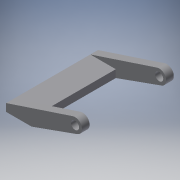
# Autodesk Inventor part: FiberMount
Saved by Autodesk Inventor 2019 (Build 230136000, 136)
## iProperties
Created: 2019-05-24
Part Number: FiberMount
Material: Generic
Document SubType Name: Modeling
Designer: aorfi
Density: 1 g/cm^3
Appearance: Default
Author: aorfi
Autodesk Inventor part; units mm, degrees
ref_plane "YZ Plane" through (0, 0, 0) normal (1, 0, 0) x (0, 1, 0)
ref_plane "XZ Plane" through (0, 0, 0) normal (0, 1, 0) x (-1, 0, 0)
ref_plane "XY Plane" through (0, 0, 0) normal (0, 0, 1) x (1, 0, 0)
sketch "Sketch1" plane through (0, 0, 0) normal (0, 1, 0) x (-1, 0, 0)
  line L0 (-5, 15) -> (5, 15)
  line L1 (5, 15) -> (5, -15)
  line L2 (5, -15) -> (-5, -15)
  line L3 (-5, -15) -> (-5, 15)
  line L4 (-5, 15) -> (5, -15) construction
  line L5 (5, 15) -> (-5, -15) construction
  point P0 (0, 0)
  dimension "d0" = 30
  dimension "d1" = 10
  constraints: 12 end point, 2 midpoint, 2 parallel, 1 horizontal, 1 perpendicular
  measures "d0" distance of L0.end L1.end
  measures "d1" distance of L1.end L2.end
extrude "Extrusion1" add sketch "Sketch1" along normal mid plane 3
sketch "Sketch2" plane through (-5, 1.5, 15) normal (0, 0, 1) x (1, 0, 0)
  circle A0 centre (27, 6) radius 1.5875
  circle A1 centre (27, 6) radius 2.75
  line L0 (26.1395, 8.6119) -> (0, 0)
  line L1 (10, -3) -> (10, 0) projected
  line L2 (10, -3) -> (27.926, 3.4106)
  line L3 (10, -3) -> (0, -3) projected
  line L4 (0, 0) -> (0, -3) projected
  point P0 (5, -1.5)
  dimension "d4" = 3.175
  dimension "d5" = 5.5
  dimension "d6" = 9
  dimension "d7" = 17
  constraints: 4 end point, 2 centre point, 2 coincident, 2 point on circle, 2 tangent
  measures "d4" diameter of A0
  measures "d5" diameter of A1
  measures "d6" distance from line of A0.centre L3
  measures "d7" distance from line of A0.centre L1
extrude "Extrusion2" add sketch "Sketch2" along normal blind 3
mirror "Mirror1" about plane through (0, 0, 0) normal (0, 0, 1) of "Extrusion2"
body "Solid1"
